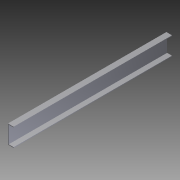
# Autodesk Inventor part: frame 7 outside U
Saved by Autodesk Inventor 2012 (Build 160160000, 160)
## iProperties
Created: 2013-08-24
Part Number: frame 7 outside U
Material: Default
Document SubType Name: Modeling
Designer: Bryce
Density: 1 g/cm^3
Author: Bryce
Autodesk Inventor part; units mm, degrees
ref_plane "YZ Plane" through (0, 0, 0) normal (1, 0, 0) x (0, 1, 0)
ref_plane "XZ Plane" through (0, 0, 0) normal (0, 1, 0) x (-1, 0, 0)
ref_plane "XY Plane" through (0, 0, 0) normal (0, 0, 1) x (1, 0, 0)
sketch "Sketch1" plane through (0, 0, 0) normal (0, 0, 1) x (1, 0, 0)
  line L0 (0, 0) -> (25.4, 0)
  line L1 (25.4, 0) -> (25.4, 3.175)
  line L2 (3.175, 82.55) -> (0, 82.55)
  line L3 (0, 82.55) -> (0, 0)
  line L4 (3.175, 79.375) -> (3.175, 3.175)
  line L5 (3.175, 3.175) -> (25.4, 3.175)
  line L6 (3.175, 82.55) -> (25.4, 82.55)
  line L7 (25.4, 82.55) -> (25.4, 79.375)
  line L8 (25.4, 79.375) -> (3.175, 79.375)
  dimension "d0" = 82.55
  dimension "d1" = 25.4
  dimension "d2" = 3.175
  dimension "d3" = 3.175
  dimension "d6" = 3.175
  dimension "d7" = 25.4
  constraints: 18 end point, 3 parallel, 2 horizontal, 2 perpendicular
  measures "d0" distance of L2.end L0.start
  measures "d1" distance of L0.start L0.end
  measures "d2" distance between parallel lines of L0 L5
  measures "d3" distance between parallel lines of L3 L4
  measures "d6" distance between parallel lines of L6 L8
  measures "d7" distance of L6.end L2.end
extrude "Extrusion1" add sketch "Sketch1" along normal blind 711.2
equation "\"d3\" = d2"
equation "\"d6\" = d3"
equation "\"d7\" = d1"
body "Solid1"
